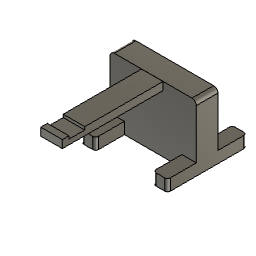
4120-Project-Testing-Stand_revised v2 (Autodesk Fusion 360 design; units mm, degrees)
Autodesk Fusion 360 part; units mm, degrees
note: some values were not read from the file. Set by a fixed rule: which sketch regions a step uses.
sketch "Sketch1" plane through (0, 0, 0) normal (0, 0, 1) x (1, 0, 0)
  line L0 (-20, 40) -> (-19.9999, 40)
  line L1 (-19.9999, 10) -> (-20, 10)
  line L2 (-20, 40) -> (40, 40)
  line L3 (40, 40) -> (40, 25)
  line L4 (40, 25) -> (-20, 25)
  line L5 (-20, 25) -> (-20, 40)
  line L6 (20, 40) -> (40, 40)
  dimension "d12" = 60
  constraint horizontal L0
  constraint horizontal L1
  constraint horizontal L2
  constraint vertical L3
  constraint horizontal L4
  constraint vertical L5
  constraint horizontal L6
  constraint coincident L2 L6.start
  measures "d12" distance of L0.start L2.end
extrude "Extrude6" add sketch "Sketch1" along normal blind 40
sketch "Sketch5" plane through (0, 25, 0) normal (0, -1, 0) x (1, 0, 0)
  line L0 (-20, 0) -> (40, 0)
  line L1 (40, 0) -> (40, 40)
  line L2 (40, 40) -> (-20, 40)
  line L3 (-20, 40) -> (-20, 0)
  line L4 (1.8726, 40) -> (16.8726, 40)
  line L5 (16.8726, 40) -> (16.8726, 45.446)
  line L6 (16.8726, 45.446) -> (1.8726, 45.446)
  line L7 (1.8726, 45.446) -> (1.8726, 40)
  point P0 (10, 40)
  dimension "d29" = 15
  constraint midpoint L2 P0
  constraint horizontal L4
  constraint vertical L5
  constraint horizontal L6
  constraint vertical L7
  constraint coincident L2 L4.start
  measures "d29" distance of L4.start L4.end
extrude "Extrude7" add sketch "Sketch5" along normal blind 70 contours L2 L4 L5 L6 L7
sketch "Sketch6" plane through (0, 0, 40) normal (0, 0, -1) x (-1, 0, 0)
  line L0 (20, 40) -> (20, 25)
  line L1 (20, 25) -> (-1.8726, 25)
  line L2 (-40, 25) -> (-40, 40)
  line L3 (-40, 40) -> (20, 40)
  line L4 (-1.8726, 25) -> (-16.8726, 25)
  line L5 (-16.8726, 25) -> (-40, 25)
extrude "Extrude8" add sketch "Sketch6" against normal blind 5.5
sketch "Sketch7" plane through (0, 25, 0) normal (0, -1, 0) x (1, 0, 0)
  line L0 (-20, 45.5) -> (-20, 0)
  line L1 (-20, 0) -> (40, 0)
  line L2 (40, 0) -> (40, 45.5)
  line L3 (-20, 8) -> (-10, 8)
  line L4 (-10, 8) -> (-10, 0)
  line L5 (-10, 0) -> (-20, 0)
  line L6 (-20, 0) -> (-20, 8)
  line L7 (30, 8) -> (40, 8)
  line L8 (40, 8) -> (40, 0)
  line L9 (40, 0) -> (30, 0)
  line L10 (30, 0) -> (30, 8)
  line L11 (16.8726, 45.446) -> (16.8726, 40)
  line L12 (1.8726, 40) -> (1.8726, 45.446)
  line L13 (40, 45.5) -> (-20, 45.5)
  line L14 (16.8726, 40) -> (1.8726, 40)
  line L15 (1.8726, 45.446) -> (16.8726, 45.446)
  dimension "d25" = 10
  dimension "d26" = 8
  dimension "d27" = 10
  dimension "d28" = 8
  constraint horizontal L3
  constraint vertical L4
  constraint horizontal L5
  constraint vertical L6
  constraint coincident L1 L4.end
  constraint coincident L0 L3.start
  constraint horizontal L7
  constraint vertical L8
  constraint horizontal L9
  constraint vertical L10
  constraint coincident L1.end L2.start
  measures "d25" distance of L3.start L3.end
  measures "d26" distance of L3.start L0.end
  measures "d27" distance of L7.start L7.end
  measures "d28" distance of L7.start L9.end
extrude "Extrude9" add sketch "Sketch7" along normal blind 20 contours L0 L1 L3 L4 L5 L6 | L1 L2 L7 L8 L9 L10
sketch "Sketch8" plane through (0, 40, 0) normal (0, 1, 0) x (-1, 0, 0)
  line L0 (-40, 0) -> (20, 0)
  line L1 (20, 0) -> (20, 45.5)
  line L2 (-40, 45.5) -> (-40, 0)
  line L3 (-40, 8) -> (-30, 8)
  line L4 (-30, 8) -> (-30, 0)
  line L5 (-30, 0) -> (-40, 0)
  line L6 (-40, 0) -> (-40, 8)
  line L7 (10, 8) -> (20, 8)
  line L8 (20, 8) -> (20, 0)
  line L9 (20, 0) -> (10, 0)
  line L10 (10, 0) -> (10, 8)
  line L11 (20, 45.5) -> (-40, 45.5)
  dimension "d34" = 10
  dimension "d35" = 8
  dimension "d36" = 8
  dimension "d37" = 10
  constraint horizontal L3
  constraint vertical L4
  constraint horizontal L5
  constraint vertical L6
  constraint coincident L0 L4.end
  constraint coincident L2 L3.start
  constraint horizontal L7
  constraint vertical L8
  constraint horizontal L9
  constraint vertical L10
  constraint coincident L0.end L1.start
  measures "d34" distance of L3.start L3.end
  measures "d35" distance of L3.start L0.start
  measures "d36" distance of L7.end L0.end
  measures "d37" distance of L7.start L7.end
extrude "Extrude10" add sketch "Sketch8" along normal blind 20 contours L0 L2 L3 L4 L5 L6 | L0 L1 L7 L8 L9 L10
sketch "Sketch10" plane through (0, 0, 45.446) normal (0, 0, 1) x (-1, 0, 0)
  line L0 (-1.8726, -25) -> (-1.8726, 45)
  line L1 (-1.8726, 45) -> (-16.8726, 45)
  line L2 (-16.8726, 45) -> (-16.8726, -25)
  line L3 (-16.8726, 40.4277) -> (-1.8726, 40.4277)
  line L4 (-1.8726, 40.4277) -> (-1.8726, 29.4277)
  line L5 (-1.8726, 29.4277) -> (-16.8726, 29.4277)
  line L6 (-16.8726, 29.4277) -> (-16.8726, 40.4277)
  line L7 (-16.8726, -25) -> (-1.8726, -25)
  dimension "d38" = 11
  constraint horizontal L3
  constraint vertical L4
  constraint horizontal L5
  constraint vertical L6
  constraint coincident L0 L4.end
  constraint coincident L2 L3.start
  measures "d38" distance of L3.start L5.end
extrude "Extrude12" cut sketch "Sketch10" against normal blind 2 contours L0 L2 L3 L4 L5 L6
fillet "Fillet1" radius 3 2 edges at (40, 32.5, 45.5) (-20, 32.5, 45.5)
fillet "Fillet2" radius 2 8 edges at (40, 5, 4) (30, 5, 4) (40, 60, 4) (-10, 5, 4) (30, 60, 4) (-10, 60, 4) (-20, 60, 4) (-20, 5, 4)
